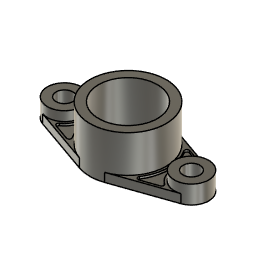
Flanged Base (Autodesk Fusion 360 design; units mm, degrees)
Autodesk Fusion 360 part; units mm, degrees
note: some values were not read from the file. Set by a fixed rule: which sketch regions a step uses.
sketch "Sketch1" plane through (0, 0, 0) normal (0, 0, 1) x (1, 0, 0)
  circle A0 centre (0, 0) radius 40.5
  circle A1 centre (0, 0) radius 52.5
  circle A2 centre (-87.5, 0) radius 11.665
  circle A3 centre (-87.5, 0) radius 23.665
  line L0 (0, 85) -> (0, -75)
  circle A4 centre (87.5, 0) radius 23.665
  circle A5 centre (87.5, 0) radius 11.665
  line L1 (-95.2986, 22.3431) -> (-17.301, 49.5674)
  line L2 (-95.2986, -22.3431) -> (-17.301, -49.5674)
  line L3 (-71.8093, 27.3643) -> (-49.826, 35.0373)
  line L4 (-71.8093, -27.3643) -> (-49.826, -35.0373)
  arc A6 (-72.5075, -22.051) -> (-72.5075, 22.051) centre (-87.5, 0) ccw
  arc A7 (-46.3329, 30.5534) -> (-46.3329, -30.5534) centre (0, 0) ccw
  arc A8 (-71.8093, 27.3643) -> (-72.5075, 22.051) centre (-70.8207, 24.5319) ccw
  arc A9 (-46.3329, 30.5534) -> (-49.826, 35.0373) centre (-48.8374, 32.2049) ccw
  arc A10 (-49.826, -35.0373) -> (-46.3329, -30.5534) centre (-48.8374, -32.2049) ccw
  arc A11 (-72.5075, -22.051) -> (-71.8093, -27.3643) centre (-70.8207, -24.5319) ccw
  line L5 (95.2986, -22.3431) -> (17.301, -49.5674)
  arc A12 (49.826, 35.0373) -> (46.3329, 30.5534) centre (48.8374, 32.2049) ccw
  arc A13 (71.8093, -27.3643) -> (72.5075, -22.051) centre (70.8207, -24.5319) ccw
  line L6 (71.8093, 27.3643) -> (49.826, 35.0373)
  arc A14 (46.3329, -30.5534) -> (46.3329, 30.5534) centre (0, 0) ccw
  circle A15 centre (87.5, 0) radius 11.665
  line L7 (71.8093, -27.3643) -> (49.826, -35.0373)
  arc A16 (46.3329, -30.5534) -> (49.826, -35.0373) centre (48.8374, -32.2049) ccw
  circle A17 centre (87.5, 0) radius 23.665
  arc A18 (72.5075, 22.051) -> (72.5075, -22.051) centre (87.5, 0) ccw
  line L8 (95.2986, 22.3431) -> (17.301, 49.5674)
  arc A19 (72.5075, 22.051) -> (71.8093, 27.3643) centre (70.8207, 24.5319) ccw
  dimension "d1" = 105
  dimension "d2" = 12
  dimension "d3" = 23.33
  dimension "d4" = 12
  dimension "d5" = 175
  dimension "d6" = 3
  dimension "d7" = 3
  dimension "d8" = 3
  dimension "d9" = 3
  dimension "d10" = 3
  dimension "d11" = 3
  dimension "d12" = 3
  constraint coincident A0.centre A1.centre
  constraint concentric A0 A1
  constraint concentric A2 A3
  constraint vertical L0
  constraint symmetric A2 L0 A5
  constraint symmetric A3 L0 A4
  constraint coincident A0.centre L0
  constraint horizontal A0.centre A2.centre
  constraint coincident A3 L1.start
  constraint coincident A1 L1.end
  constraint coincident A3 L2.start
  constraint coincident A1 L2.end
  constraint tangent A3 L1
  constraint tangent A1 L1
  constraint tangent A3 L2
  constraint tangent A1 L2
  constraint concentric A3 A6
  constraint parallel L1 L3
  constraint parallel L2 L4
  constraint tangent L3 A8
  constraint tangent A6 A8
  constraint tangent L3 A9
  constraint tangent A7 A9
  constraint equal A8 A9
  constraint tangent L4 A10
  constraint tangent A7 A10
  constraint tangent L4 A11
  constraint tangent A6 A11
  constraint symmetric A2 L0 A15
  constraint symmetric A3 L0 A17
  constraint symmetric L0 L1.start L8.start
  constraint symmetric L0 L1.end L8.end
  constraint symmetric L0 L2.start L5.start
  constraint symmetric L0 L2.end L5.end
  constraint symmetric L0 A6 A18
  constraint symmetric L0 A7 A14
  constraint symmetric L0 L3.start L6.start
  constraint symmetric L0 A6.end A18.start
  constraint symmetric L0 A8 A19
  constraint symmetric L0 L3.end A12.start
  constraint symmetric L0 A7.start A12.end
  constraint symmetric L0 A9 A12
  constraint symmetric L0 L4.end L7.end
  constraint symmetric L0 A7.end A14.start
  constraint symmetric L0 A10 A16
  constraint symmetric L0 L4.start A13.start
  constraint symmetric L0 A6.start A13.end
  constraint symmetric L0 A11 A13
  measures "d1" diameter of A1
  measures "d2" distance of A0 A1
  measures "d3" diameter of A2
  measures "d4" distance of A2 A3
  measures "d5" distance of A2.centre A4.centre
  measures "d6" distance of A3 A6
  measures "d7" distance of A1 A7
  measures "d8" distance of L1 L3
  measures "d9" distance of L2 L4
  measures "d10" radius of A8
  measures "d11" radius of A10
  measures "d12" radius of A11
extrude "Extrude1" add sketch "Sketch1" along normal blind 38 contours A0 A1 L0 | A0 A1 L0 makes body 1
sketch "Sketch2" plane through (0, 0, 0) normal (0, 0, 1) x (1, 0, 0)
  circle A0 centre (87.5, 0) radius 11.665
  circle A1 centre (87.5, 0) radius 23.665
  line L0 (0, 67.4861) -> (0, -70)
  line L1 (0, 67.4861) -> (0, -70)
  circle A2 centre (-87.5, 0) radius 23.665
  circle A3 centre (-87.5, 0) radius 11.665
  dimension "d15" = 23.33
  dimension "d16" = 12
  dimension "d17" = 175
  constraint concentric A0 A1
  constraint horizontal origin A0.centre
  constraint vertical L0
  constraint symmetric A0 L0 A3
  constraint symmetric A1 L0 A2
  constraint symmetric L1.start L0 L0.start
  constraint symmetric L1.end L0 L0.end
  constraint vertical origin L0.start
  measures "d15" diameter of A0
  measures "d16" distance of A0 A1
  measures "d17" distance of A0.centre A2.centre
extrude "Extrude2" add sketch "Sketch2" along normal blind 25 separate body makes body 2 at (111.0474, -2.3563, 8.3333) makes body 3 at (-63.9526, -2.3563, 8.3333)
extrude "Extrude3" add 1 faces at (-19.7228, 44.199, 38) along direction (0, 0, 1) blind 25 on bodies 1 bodies 1
sketch "Sketch3" plane through (0, 0, 0) normal (0, 0, 1) x (1, 0, 0)
  circle A0 centre (-87.5, 0) radius 23.665
  circle A1 centre (0, 0) radius 52.5
  line L0 (-95.2986, 22.3431) -> (-17.301, 49.5674)
  line L1 (-95.2986, -22.3431) -> (-17.301, -49.5674)
  line L2 (0, 66.8744) -> (0, -68.3016)
  line L3 (95.2986, 22.3431) -> (17.301, 49.5674)
  line L4 (95.2986, -22.3431) -> (17.301, -49.5674)
  circle A2 centre (87.5, 0) radius 23.665
  constraint coincident A0 L0.start
  constraint coincident A1 L0.end
  constraint tangent A0 L0
  constraint tangent A1 L0
  constraint coincident A0 L1.start
  constraint coincident A1 L1.end
  constraint tangent A1 L1
  constraint tangent A0 L1
  constraint vertical L2
  constraint symmetric L0.start L2 L3.start
  constraint symmetric L0.end L2 L3.end
  constraint symmetric L1.start L2 L4.start
  constraint symmetric L1.end L2 L4.end
  constraint tangent L3 A2
extrude "Extrude4" add sketch "Sketch3" along normal blind 12 contours A0 A1 L0 L1 | A1 L3 L4 A2 bodies 1 2 3
sketch "Sketch4" plane through (0, 0, 12) normal (0, 0, 1) x (-1, 0, 0)
  arc A0 (-95.2986, -22.3431) -> (-95.2986, 22.3431) centre (-87.5, 0) ccw
  line L0 (-95.2986, -22.3431) -> (-17.301, -49.5674)
  arc A1 (-17.301, 49.5674) -> (-17.301, -49.5674) centre (0, 0) ccw
  line L1 (-17.301, 49.5674) -> (-95.2986, 22.3431)
  line L2 (-71.8093, 27.3643) -> (-49.826, 35.0373)
  line L3 (-71.8093, -27.3643) -> (-49.826, -35.0373)
  arc A2 (-72.5075, -22.051) -> (-72.5075, 22.051) centre (-87.5, 0) ccw
  arc A3 (-46.3329, 30.5534) -> (-46.3329, -30.5534) centre (0, 0) ccw
  arc A4 (-71.8093, 27.3643) -> (-72.5075, 22.051) centre (-70.8207, 24.5319) ccw
  arc A5 (-46.3329, 30.5534) -> (-49.826, 35.0373) centre (-48.8374, 32.2049) ccw
  arc A6 (-49.826, -35.0373) -> (-46.3329, -30.5534) centre (-48.8374, -32.2049) ccw
  arc A7 (-72.5075, -22.051) -> (-71.8093, -27.3643) centre (-70.8207, -24.5319) ccw
  line L4 (0, 70) -> (0, -73.9622)
  arc A8 (49.826, 35.0373) -> (46.3329, 30.5534) centre (48.8374, 32.2049) ccw
  arc A9 (72.5075, 22.051) -> (72.5075, -22.051) centre (87.5, 0) ccw
  arc A10 (72.5075, 22.051) -> (71.8093, 27.3643) centre (70.8207, 24.5319) ccw
  arc A11 (46.3329, -30.5534) -> (49.826, -35.0373) centre (48.8374, -32.2049) ccw
  arc A12 (71.8093, -27.3643) -> (72.5075, -22.051) centre (70.8207, -24.5319) ccw
  line L5 (71.8093, -27.3643) -> (49.826, -35.0373)
  arc A13 (46.3329, -30.5534) -> (46.3329, 30.5534) centre (0, 0) ccw
  line L6 (71.8093, 27.3643) -> (49.826, 35.0373)
  dimension "d24" = 3
  dimension "d25" = 3
  dimension "d26" = 3
  dimension "d27" = 3
  dimension "d28" = 3
  dimension "d29" = 3
  dimension "d30" = 3
  dimension "d31" = 3
  constraint concentric A0 A2
  constraint coincident A1.centre A3.centre
  constraint parallel L1 L2
  constraint parallel L0 L3
  constraint tangent L2 A4
  constraint tangent A2 A4
  constraint tangent L2 A5
  constraint tangent A3 A5
  constraint tangent L3 A6
  constraint tangent A3 A6
  constraint tangent L3 A7
  constraint tangent A2 A7
  constraint vertical L4
  constraint symmetric A2 L4 A9
  constraint symmetric A3 L4 A13
  constraint symmetric L2.start L4 A10.end
  constraint symmetric A2.end L4 A9.start
  constraint symmetric A4 L4 A10
  constraint symmetric L2.end L4 A8.start
  constraint symmetric A3.start L4 A8.end
  constraint symmetric A5 L4 A8
  constraint symmetric L3.end L4 A11.end
  constraint symmetric A3.end L4 A11.start
  constraint symmetric A6 L4 A11
  constraint symmetric L3.start L4 A12.start
  constraint symmetric A2.start L4 A9.end
  constraint symmetric A7 L4 A12
  measures "d24" distance of A0 A2
  measures "d25" distance of A1 A3
  measures "d26" distance of L1 L2
  measures "d27" distance of L0 L3
  measures "d28" radius of A4
  measures "d29" radius of A5
  measures "d30" radius of A6
  measures "d31" radius of A7
extrude "Extrude5" cut sketch "Sketch4" against normal blind 3 contours L2 L3 A2 A3 A4 A5 A6 A7 | A8 A9 A10 A11 A12 L5 A13 L6 bodies 1
